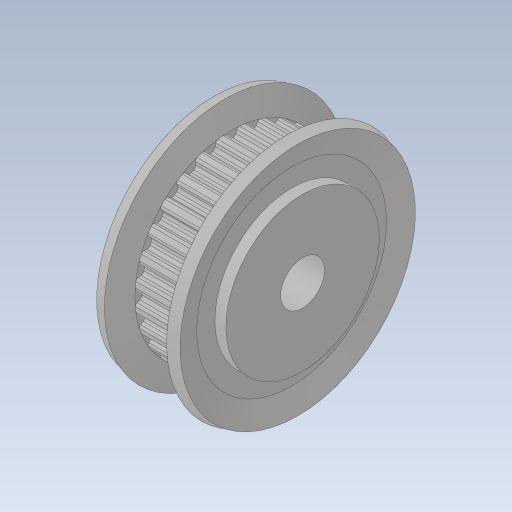
# Autodesk Inventor part: ATP28MXL013-A-H4_b
Saved by Autodesk Inventor 2024 (Build 280153000, 153)
## iProperties
Category: PARTsolutions
Company: MISUMI
Created: 2023-09-11
Part Number: ATP28MXL013-A-H4_b
Material: Generic
Catalog Web Link: www.cadenas.de
Description: ATP__MXL013, ATP__MXL019, ATP__MXL025, ATP__MXL037, ATP__MXL050, BTP__MXL013, BTP__MXL019, BTP__MXL025, BTP__MXL037, BTP__MXL050, KTP__MXL013, KTP__MXL019, KTP__MXL025, KTP__MXL037, KTP__MXL050, NTP__MXL013, NTP__MXL019, NTP__MXL025, NTP__MXL037, NTP__MXL050, MTP__MXL025, MTP__MXL037, MTPB__MXL025, MTPB__MXL037, MTPP__MXL025, MTPP__MXL037, STP__MXL013, STP__MXL019, STP__MXL025, STP__MXL037, STP__MXL050, KATP__MXL013, KATP__MXL019, KATP__MXL025, KATP__MXL037, KATP__MXL050, KKTP__MXL013, KKTP__MXL019, KKTP__MXL025, KKTP__MXL037, KKTP__MXL050_body-Timing Pulleys MXL Type
Vendor: MISUMI
Document SubType Name: Modeling
Designer: psAdmin
Manufacturer: MISUMI
Mass: 1.9758 g
Surface Area: 16.8784 cm^2
Volume: 1.9758 cm^3
Density: 1 g/cm^3
Appearance: PSOLRGB-175-175-175
PSOL_IDENT_0: {$CADENAS_DATA/23d-libs/misumi/metric/51_timing_pulleys/mtp_mxl/atp_mxl.prj},968 {VTYP=3D},{NB=ATP28
PSOL_IDENT_1: MXL013-A-H4_b},{LINA=ATP28MXL013-A-H4},{NN=ATP__MXL013, ATP__MXL019, ATP__MXL025, ATP__MXL037, ATP__
PSOL_IDENT_2: MXL050, BTP__MXL013, BTP__MXL019, BTP__MXL025, BTP__MXL037, BTP__MXL050, KTP__MXL013, KTP__MXL019, K
PSOL_IDENT_3: TP__MXL025, KTP__MXL037, KTP__MXL050, NTP__MXL013, NTP__MXL019, NTP__MXL025, NTP__MXL037, NTP__MXL05
PSOL_IDENT_4: 0, MTP__MXL025, MTP__MXL037, MTPB__MXL025, MTPB__MXL037, MTPP__MXL025, MTPP__MXL037, STP__MXL013, ST
PSOL_IDENT_5: P__MXL019, STP__MXL025, STP__MXL037, STP__MXL050, KATP__MXL013, KATP__MXL019, KATP__MXL025, KATP__MX
PSOL_IDENT_6: L037, KATP__MXL050, KKTP__MXL013, KKTP__MXL019, KKTP__MXL025, KKTP__MXL037, KKTP__MXL050_body},{DATE=
PSOL_IDENT_7: 06.01.2023 09:01:29},{GEOMDATE=06.01.2023 09:01:06},{VERSION=},{LINEID=350},{WBVAR=MATP,ST,TNW,PS,SB
PSOL_IDENT_8: S,DD,Z,J,Q,R,S,T,ALT1,ALT2,M,QSC,QFC,QTC,ALT3,K,KSC,KFC,KTC,ALT4,ZM,ZSC,ZFC,ZTC,ALT5,ALT6,ALT7,FC,AL
PSOL_IDENT_9: T8,SRG,ALT9,BTC,TL,ALT10,TPC,ALT11,BC,ALT12,SLH,ALT13,BN},{WBNUMERIC=DD,Z,J,Q,R,S,T,QSC,QFC,QTC,K,KS
PSOL_IDENT_10: C,KFC,KTC,ZSC,ZFC,ZTC,FC,SRG,BTC,TL,BC,SLH,BN}  {NB=ATP28MXL013-A-H4_b},{LINA=ATP28MXL013-A-H4},{KT=
PSOL_IDENT_11: DUMMY},{PN=ATP28MXL013-A-H4},{TYPE=ATP},{MATP=A2017},{MATPALG= 'A2017','Aluminum Alloy 2000 series','
PSOL_IDENT_12: S45C','1045 Carbon Steel Equivalent','SUS304','SUS304', 'A6000', '6000 Series Aluminum Alloy' },{ST=
PSOL_IDENT_13: CA},{STALG= 'CA','Clear Anodize','BA','Black Anodize','HAT','Hard Clear Anodize','ENP','Electroless
PSOL_IDENT_14: Nickel Plating' },{NT=28},{TNW=MXL013},{TNWALG= 'MXL013','MXL019','MXL025','MXL037','MXL050' },{BW=3
PSOL_IDENT_15: .2mm (1/8inch)},{PS=A},{PSALG= 'A','B' },{SBS=H},{SBSALG= 'H','Round Hole','V','Stepped Hole' },{DD=
PSOL_IDENT_16: 4.00},{DDALG=[4:4/1],4.5,[5:6/1],6.35,[7:10/1]},{DDHA=[4:4/1],4.5,[5:6/1],6.35,[7:10/1]},{DDNA=},{DD
PSOL_IDENT_17: NK=[10:10/1]},{DDCA=},{DDVA=[4:4/1],4.5,[5:6/1],6.35,[7:8/1]},{DDY=[4:8/1]},{DDWB=[4:6/1]},{DDHBK=},
PSOL_IDENT_18: {DDPBK=},{DDNB=},{DDCB=},{DDVFB=},{Z=0},{ZALG=[0]},{ZMIN=6.000},{ZAMAX=10.000},{ZBMAX=0.000},{DDZ=4.
PSOL_IDENT_19: 000},{J=0.0},{JALG=[0]},{JMIN=2.000},{JMAX=6.500},{JPN=},{Q=0},{QALG=[0]},{QRMIN=6.000},{QRMAX=10},{
PSOL_IDENT_20: WBQMIN=8.000},{R=0},{RALG=[0]},{WBRMAX=-2.000},{S=0.0},{SALG=[0]},{SMAX=2.5},{T=0.0},{TALG=[0]},{TMA
PSOL_IDENT_21: X=5.5},{SBSPN=-H4},{A=4.5},{W=8.5},{L=0.0},{PD=18.11},{OD=17.60},{D=0},{DALG=12.000},{DE=14},{F=22},
PSOL_IDENT_22: {E=14},{TT=1.0},{BBK=0.000},{TTK=0.0},{ALT1=},{ALT1ALG= '','Not applicable' },{ANG=115.714},{ALT1PN=
PSOL_IDENT_23: },{ALT2=},{ALT2ALG= '','Not applicable' },{M=N/A},{MALG= 'N/A' },{MFTALG= 'N/A' },{MSALG= 'N/A' },{M
PSOL_IDENT_24: 3D=0.000},{KDML=0.000},{ML=0.000},{MUL=0.000},{PITCH=0.000},{QSC=0.0},{QSCALG=0},{QFC=0.0},{QFCALG=0
PSOL_IDENT_25: },{QTC=0.0},{QTCALG=0},{QPCDMIN=0.000},{QPCDMINALG=0.000},{QPCDMAX=10.000},{ALT2PN=},{TAP=0.000},{AL
PSOL_IDENT_26: T3=},{ALT3ALG= '','Not applicable' },{K=0.0},{KALG=0},{KMIN=4.000},{KFTMAX=0.000},{KSMAX=0.000},{KSC=
PSOL_IDENT_27: 0.0},{KSCALG=0},{KFC=0.0},{KFCALG=0},{KTC=0.0},{KTCALG=0},{KSCMIN=8.000},{KPCDMIN=8.000},{KPCDMINALG=
PSOL_IDENT_28: 8.000},{KPCDMAX=10.000},{ALT3PN=},{ALT4=},{ALT4ALG= '','Not applicable' },{ALT4MIN=14.500},{ALT4MAX=
PSOL_IDENT_29: 3.500},{ZM=N/A},{ZMALG= 'N/A' },{ZMFTALG= 'N/A' },{ZMSALG= 'N/A' },{ZMDD1=0.0},{ZMDD2=0.0},{ZMHH=0.0
PSOL_IDENT_30: },{ZSC=0.0},{ZSCALG=[0]},{ZFC=0.0},{ZFCALG=[0]},{ZTC=0.0},{ZTCALG=[0]},{ZPCDMIN=0.000},{ZPCDMINALG=0
PSOL_IDENT_31: .000},{ZPCDMAX=10.000},{ALT4PN=},{ALT5=},{ALT5ALG= '','w/o Flange not Attached','NFC','with NFC (Fla
PSOL_IDENT_32: nge not Attached)' },{ALT5PN=},{ALT6=},{ALT6ALG= '','w/o Flange Attached on One Side Only','RFC','wi
PSOL_IDENT_33: th RFC (Flange Attached on The Boss Side Only)','LFC','with LFC (Flange Attached on The Opposite Sid
PSOL_IDENT_34: e Only)' },{ALT6PN=},{ALT7=},{ALT7ALG= '','w/o FC (Flange Cut)','FC','with FC (Flange Cut)' },{FC=0.
PSOL_IDENT_35: 0},{FCALG=0},{FCMIN=19.0},{FCMAX=20.0},{ALT7PN=},{ALT8=},{ALT8ALG= '','Not applicable' },{ALT8ALGALG=
PSOL_IDENT_36: 10.000},{ALT8DD2=0.000},{ALT8MM=0.000},{ALT8NN=0.000},{QC=0.000},{KC=0.000},{ZC=0.000},{SRG=0.0},{SR
PSOL_IDENT_37: GALG=[0]},{SRGMAX=0.0},{SRGMAX1=0.000},{DD2=0.0},{MM=0.00},{NN=0.00},{ALT8PN=},{ALT9=},{ALT9ALG= '','
PSOL_IDENT_38: w/o BTC (Taper for Bearing Holder)','BTC','with BTC (Taper for Bearing Holder)' },{BTC9=6.000},{TL9=
PSOL_IDENT_39: 1.000},{BTC=0},{BTCALG=[0]},{TL=0.0},{TLALG=0},{TLMIN=1.000},{TLMAX=-9.000},{BTCL=0},{BTCD=0},{ALT9P
PSOL_IDENT_40: N=},{WLBCTL=8.500},{ALT10=},{ALT10ALG= '','Not applicable' },{TPC=N/A},{TPCALG= 'N/A' },{TPCM=3.000}
PSOL_IDENT_41: ,{ALT10PN=},{ALT11=},{ALT11ALG= '','Not applicable' },{BC=0.0},{BCALG=0},{BCMIN=3},{BCMAX=-9},{M1WBC=
PSOL_IDENT_42: 4.25},{ALT11PN=},{KTT=6.8},{ALT12=},{ALT12ALG= '','Not applicable' },{SLH=0},{SLHALG=[0]},{ALT12PN=}
PSOL_IDENT_43: ,{ALT13=},{ALT13ALG= '', 'Not applicable' },{BN=0.0},{BNALG=0},{BNMIN=-8},{BNMAX=1.5},{ALT13PN=},{AC=
PSOL_IDENT_44: -},{M1=3.000},{M1L=3.000},{TEDEG=20.000},{TEB=0.670},{CD=0}
NB: ATP28MXL013-A-H4_b
NN: 0
NT: 28
NBSYN: $PN._b
LINA: ATP28MXL013-A-H4
CATALOG: Misumi
PN: ATP28MXL013-A-H4
MATP: Aluminum Alloy 2000 series
ST: Clear Anodize
TNW: MXL013
BW: 3.2mm (1/8inch)
PS: A
SBS: Round Hole
DD: 4
Z: 0
J: 0
Q: 0
R: 0
S: 0
T: 0
A: 4.5
W: 8.5
L: 0
PD: 18.11
OD: 17.6
D: 0
F: 22
E: 14
ALT1: Not applicable
ALT2: Not applicable
M: N/A
QSC: 0
QFC: 0
QTC: 0
ALT3: Not applicable
K: 0
KSC: 0
KFC: 0
KTC: 0
ALT4: Not applicable
ZM: N/A
ZMDD1: 0
ZMDD2: 0
ZMHH: 0
ZSC: 0
ZFC: 0
ZTC: 0
ALT5: w/o Flange not Attached
ALT6: w/o Flange Attached on One Side Only
ALT7: w/o FC (Flange Cut)
FC: 0
ALT8: Not applicable
SRG: 0
DD2: 0
MM: 0
ALT9: w/o BTC (Taper for Bearing Holder)
BTC: 0
TL: 0
BTCL: 0
BTCD: 0
ALT10: Not applicable
TPC: N/A
ALT11: Not applicable
BC: 0
ALT12: Not applicable
SLH: 0
ALT13: Not applicable
BN: 0
AC: -
SUPPLIER: MISUMI
ARTICLENO: ATP28MXL013-A-H4_b
BOMINFO: ATP28MXL013-A-H4
CREATOR: CADENAS GmbH
Title: ATP28MXL013-A-H4
Author: Cadenas PARTsolutions
Comments: Timing Pulleys MXL Type
Autodesk Inventor part; units mm, degrees
note: some values were not read from the file. Chosen so that the rebuilt part matches the saved one: pattern direction of "Circular Pattern1".
ref_plane "YZ Plane" through (0, 0, 0) normal (1, 0, 0) x (0, 1, 0)
ref_plane "XZ Plane" through (0, 0, 0) normal (0, 1, 0) x (-1, 0, 0)
ref_plane "XY Plane" through (0, 0, 0) normal (0, 0, 1) x (1, 0, 0)
sketch "_____2" plane through (0, 0, 0) normal (0, 0, 1) x (1, 0, 0)
  line L0 (8.5, 0) -> (0, 0)
  line L1 (0, 0) -> (0, 7)
  line L2 (0, 7) -> (1, 7)
  line L3 (1, 7) -> (1, 8.6683)
  line L4 (1, 8.6683) -> (0.4446, 10.7412)
  line L5 (0.4446, 10.7412) -> (1.4105, 11)
  line L6 (1.4105, 11) -> (2, 8.8)
  line L7 (2, 8.8) -> (6.5, 8.8)
  line L8 (6.5, 8.8) -> (7.0895, 11)
  line L9 (7.0895, 11) -> (8.0554, 10.7412)
  line L10 (8.0554, 10.7412) -> (7.5, 8.6683)
  line L11 (7.5, 8.6683) -> (7.5, 7)
  line L12 (7.5, 7) -> (8.5, 7)
  line L13 (8.5, 7) -> (8.5, 0)
  line L14 (8.5, 0) -> (0, 0)
  constraints: 30 end point
revolve "Revolution1" add sketch "_____2" angle 360 about axis through (8.5, 0, 0) along (1, 0, 0)
sketch "Sketch2" plane through (8.5, 0, 0) normal (1, 0, 0) x (0, 0, -1)
  point P0 (0, 0)
hole "Hole1" at (8.5, 0, 0) direction (-1, 0, 0) diameter 4 depth 8.5
sketch "_____6" plane through (2, 0, 0) normal (1, 0, 0) x (0, 0, -1)
  line L0 (-0.7612, 9.0229) -> (-0.7398, 8.7688)
  arc A0 (-0.5043, 8.6183) -> (-0.7398, 8.7688) centre (-0.7205, 8.5397) ccw
  line L1 (-0.5043, 8.6183) -> (-0.409, 8.3564)
  arc A1 (-0.409, 8.3564) -> (-0.1226, 8.1591) centre (-0.1271, 8.459) ccw
  arc A2 (0.1226, 8.1591) -> (-0.1226, 8.1591) centre (0, 0) ccw
  arc A3 (0.1226, 8.1591) -> (0.409, 8.3564) centre (0.1271, 8.459) ccw
  line L2 (0.409, 8.3564) -> (0.5043, 8.6183)
  arc A4 (0.7398, 8.7688) -> (0.5043, 8.6183) centre (0.7205, 8.5397) ccw
  line L3 (0.7398, 8.7688) -> (0.7612, 9.0229)
  arc A5 (0.7612, 9.0229) -> (-0.7612, 9.0229) centre (0, 0) ccw
  constraints: 12 point on circle, 8 end point, 6 centre point
extrude "Extrusion1" cut sketch "_____6" along normal blind 4.5
pattern_circular "Circular Pattern1" count 28 over 360 about axis through (2, 0, 0) along (1, 0, 0) of "Extrusion1"
body "Solid1"
